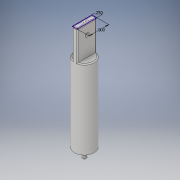
# Autodesk Inventor part: 2016.06.13 height guide
Saved by Autodesk Inventor 2017 (Build 210142000, 142)
## iProperties
Created: 2016-06-13
Part Number: 2016.06.13 height guide
Material: Generic
Document SubType Name: Modeling
Designer: Darien Morrow
Density: 1 g/cm^3
Appearance: Default
Author: Darien Morrow
Autodesk Inventor part; units mm, degrees
ref_plane "YZ Plane" through (0, 0, 0) normal (1, 0, 0) x (0, 1, 0)
ref_plane "XZ Plane" through (0, 0, 0) normal (0, 1, 0) x (-1, 0, 0)
ref_plane "XY Plane" through (0, 0, 0) normal (0, 0, 1) x (1, 0, 0)
sketch "Sketch1" plane through (0, 0, 0) normal (0, 0, 1) x (1, 0, 0)
  line L0 (0, 0) -> (12.7, 0)
  line L1 (12.7, 0) -> (12.7, 139.7)
  line L2 (12.7, 139.7) -> (0, 139.7)
  line L3 (0, 139.7) -> (0, 0)
  line L4 (0, 0) -> (2.54, 0)
  line L5 (2.54, 0) -> (2.54, -12.7)
  line L6 (2.54, -12.7) -> (0, -12.7)
  line L7 (0, -12.7) -> (0, 0)
  dimension "d0" = 12.7
  dimension "d1" = 139.7
  dimension "d2" = 12.7
  dimension "d3" = 2.54
  constraints: 16 end point, 4 parallel, 2 horizontal, 2 perpendicular
  measures "d0" distance between parallel lines of L1 L3
  measures "d1" distance between parallel lines of L0 L2
  measures "d2" distance between parallel lines of L6 L0
  measures "d3" distance between parallel lines of L5 L7
revolve "Revolution1" add sketch "Sketch1" angle 360 about axis through (0, 139.7, 0) along (0, -1, 0)
sketch "Sketch4" plane through (0, 139.7, 0) normal (0, 1, 0) x (1, 0, 0)
  line L0 (3.175, -12.7) -> (3.175, 12.7)
  line L1 (3.175, 12.7) -> (-3.175, 12.7)
  line L2 (-3.175, 12.7) -> (-3.175, -12.7)
  line L3 (-3.175, -12.7) -> (3.175, -12.7)
  line L4 (3.175, -12.7) -> (-3.175, 12.7) construction
  line L5 (3.175, 12.7) -> (-3.175, -12.7) construction
  point P0 (0, 0)
  dimension "d24" = 6.35
  dimension "d25" = 25.4
  constraints: 12 end point, 2 midpoint, 2 parallel, 1 perpendicular, 1 vertical
  measures "d24" distance between parallel lines of L0 L2
  measures "d25" distance between parallel lines of L1 L3
sketch "Sketch5" plane through (0, 139.7, 0) normal (0, 1, 0) x (1, 0, 0)
  line L0 (-3.2918, -12.7) -> (-12.7, -12.7)
  line L1 (-12.7, -12.7) -> (-12.7, 12.7)
  line L2 (-12.7, 12.7) -> (-3.2918, 12.7)
  line L3 (-3.2918, 12.7) -> (-3.2918, -12.7)
  line L4 (3.4651, -12.7) -> (12.7, -12.7)
  line L5 (12.7, -12.7) -> (12.7, 12.7)
  line L6 (12.7, 12.7) -> (3.4651, 12.7)
  line L7 (3.4651, 12.7) -> (3.4651, -12.7)
  point P0 (0, 0)
  constraints: 16 end point, 4 parallel, 2 horizontal, 2 perpendicular, 2 point on line
extrude "Extrusion2" cut sketch "Sketch5" against normal blind 38.1
sketch "Sketch6" plane through (3.4651, 139.7, 12.2181) normal (1, 0, 0) x (0, 0, -1)
  line L0 (-0.4819, -139.7) -> (24.9181, -139.7) projected
  point P0 (12.2181, -139.7)
  point P1 (12.2181, -12.7)
  dimension "d28" = 127
  measures "d28" distance from line of L0 point (12.218, -12.7)
hole "Hole2" at (3.4651, 127, 0) direction (-1, 0, 0) diameter 5.08 end through all
chamfer "Chamfer3" distance 1.27 angle 45 12 edges at (10.1316, 101.6, -7.6578) (10.1316, 101.6, 7.6578) (3.4651, 120.65, -12.2181) (3.4651, 120.65, 12.2181) (3.4651, 139.7, 0) (0.0899, 139.7, -12.6997) (0.0899, 139.7, 12.6997) (-3.2918, 139.7, 0) (-3.2918, 120.65, -12.266) (-3.2918, 120.65, 12.266) (-12.7, 101.6, 0) (-2.54, -12.7, 0)
body "Solid1"
